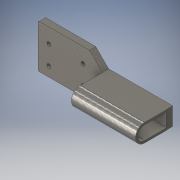
# Autodesk Inventor part: WireHolderPiece1
Saved by Autodesk Inventor 2016 (Build 200138000, 138)
## iProperties
Created: 2015-12-01
Part Number: WireHolderPiece1
Material: Generic
Document SubType Name: Modeling
Designer: Javier
Density: 1 g/cm^3
Appearance: Diamond Plate
Author: Javier
Autodesk Inventor part; units mm, degrees
ref_plane "XZ Plane" through (0, 0, 0) normal (0, 1, 0) x (-1, 0, 0)
ref_plane "XY Plane" through (0, 0, 0) normal (0, 0, 1) x (1, 0, 0)
sketch "Sketch4" plane through (0, 0, 0) normal (0, 0, 1) x (1, 0, 0)
  line L0 (-8.4948, -28.1443) -> (-8.4948, 35.8557)
  line L1 (-6.4948, 37.8557) -> (71.5052, 37.8557)
  line L2 (71.5052, 37.8557) -> (91.5052, 17.8557)
  line L3 (-6.4948, -30.1443) -> (71.5052, -30.1443)
  line L4 (71.5052, -30.1443) -> (91.5052, -10.1443)
  line L5 (91.5052, -10.1443) -> (91.5052, 17.8557)
  line L6 (91.5052, 17.8557) -> (191.5052, 17.8557)
  line L7 (191.5052, 17.8557) -> (191.5052, -10.1443)
  line L8 (191.5052, -10.1443) -> (91.5052, -10.1443)
  arc A0 (-6.4948, 37.8557) -> (-8.4948, 35.8557) centre (-6.4948, 35.8557) ccw
  arc A1 (-8.4948, -28.1443) -> (-6.4948, -30.1443) centre (-6.4948, -28.1443) ccw
  line L9 (71.5052, 37.8557) -> (91.5052, 17.8557)
  line L10 (71.5052, -30.1443) -> (91.5052, -10.1443)
  line L11 (91.5052, 17.8557) -> (91.5052, -10.1443)
  point P0 (0, 0)
  point P1 (-8.4948, -30.1443)
  point P2 (-8.4948, 37.8557)
  dimension "d7" = 68
  dimension "d8" = 80
  dimension "d9" = 80
  dimension "d10" = 135
  dimension "d11" = 135
  dimension "d12" = 20
  dimension "d13" = 20
  dimension "d14" = 28
  dimension "d15" = 2
  dimension "d16" = 2
  dimension "d19" = 100
  constraints: 24 end point, 4 point on circle, 4 point on line, 4 tangent, 3 perpendicular, 2 centre point, 2 collinear, 2 horizontal, 2 vertical
  measures "d7" distance of point (-8.495, -30.144) point (-8.495, 37.856)
  measures "d8" distance of point (-8.495, 37.856) L1.end
  measures "d9" distance of point (-8.495, -30.144) L3.end
  measures "d10" angle of L4 L3
  measures "d11" angle of L2 L1
  measures "d12" horizontal distance of L1.end L2.end
  measures "d13" horizontal distance of L3.end L4.end
  measures "d14" distance of L4.end L5.end
  measures "d15" radius of A0
  measures "d16" radius of A1
  measures "d19" distance of L6.start L6.end
extrude "Extrusion2" add sketch "Sketch4" along normal blind 10
ref_plane "Work Plane1" through (192, 0, 0) normal (1, 0, 0) x (0, 1, 0)
sketch "Sketch5" plane through (192, 0, 0) normal (1, 0, 0) x (0, 1, 0)
  line L0 (17.8557, 10) -> (17.8557, 44.45)
  line L1 (-10.1443, 0) -> (-10.1443, 10) projected
  line L2 (-10.1443, 10) -> (-10.1443, 44.45)
  arc A0 (17.8557, 44.45) -> (-10.1443, 44.45) centre (3.8557, 44.45) ccw
  line L3 (14.3557, 10) -> (14.3557, 44.45)
  line L4 (-6.6443, 10) -> (-6.6443, 44.45)
  arc A1 (14.3557, 44.45) -> (-6.6443, 44.45) centre (3.8557, 44.45) ccw
  line L5 (14.3557, 44.45) -> (14.3557, 10)
  line L6 (-6.6443, 44.45) -> (-6.6443, 10)
  line L7 (-10.1443, 10) -> (17.8557, 10) projected
  line L8 (17.8557, 10) -> (14.3557, 10)
  line L9 (-6.6443, 10) -> (-10.1443, 10)
  point P0 (0, 0)
  dimension "d21" = 34.45
  dimension "d22" = 3.5
  dimension "d23" = 3.5
  constraints: 16 end point, 4 point on circle, 4 tangent, 2 centre point, 2 vertical, 1 collinear, 1 horizontal
  measures "d21" distance of L0.start L0.end
  measures "d22" distance between parallel lines of L3 L0
  measures "d23" distance between parallel lines of L2 L4
extrude "Extrusion3" add sketch "Sketch5" against normal blind 100 contours L7 L3 A1 L4 L2 A0 L0
sketch "Sketch6" plane through (0, 0, 0) normal (0, 0, 1) x (1, 0, 0)
  line L0 (-54.1714, 0) -> (81.2571, 0)
  line L1 (8.4643, 0) -> (8.4643, 14.85)
  line L2 (8.4643, 0) -> (8.4643, -14.85)
  circle A0 centre (8.4643, 14.85) radius 3
  circle A1 centre (8.4643, -14.85) radius 3
  line L3 (61.9125, 0) -> (61.9125, 14.85)
  line L4 (61.9125, 0) -> (61.9125, -14.85)
  circle A2 centre (61.9125, 14.85) radius 3
  circle A3 centre (61.9125, -14.85) radius 3
  point P0 (0, 0)
  dimension "d26" = 14.85
  dimension "d27" = 14.85
  dimension "d28" = 6
  dimension "d29" = 6
  dimension "d30" = 14.85
  dimension "d31" = 14.85
  dimension "d32" = 6
  dimension "d33" = 6
  constraints: 10 end point, 4 centre point, 4 coincident, 2 perpendicular, 2 point on line, 2 vertical, 1 horizontal
  measures "d26" distance of L1.start L2.end
  measures "d27" distance of L1.start L1.end
  measures "d28" diameter of A0
  measures "d29" diameter of A1
  measures "d30" distance of L3.start L4.end
  measures "d31" distance of L3.start L3.end
  measures "d32" diameter of A2
  measures "d33" diameter of A3
extrude "Extrusion4" cut sketch "Sketch6" along normal blind 10
thread "Thread1" size "M6x1" class "6H" standard "ANSI Metric M Profile" full length
thread "Thread2" size "M6x1" class "6H" standard "ANSI Metric M Profile" full length
thread "Thread3" size "M6x1" class "6H" standard "ANSI Metric M Profile" full length
thread "Thread4" size "M6x1" class "6H" standard "ANSI Metric M Profile" full length
body "Solid2"
